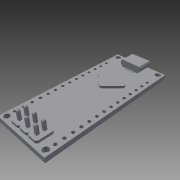
# Autodesk Inventor part: Arduino Nano
Saved by Autodesk Inventor 2015 (Build 190159000, 159)
## iProperties
Created: 2018-12-22
Part Number: Arduino Nano
Material: Типовые
Document SubType Name: Modeling
Designer: kostya
Density: 1 g/cm^3
Appearance: По умолчанию
Author: kostya
Autodesk Inventor part; units mm, degrees
ref_plane "YZ Plane" through (0, 0, 0) normal (1, 0, 0) x (0, 1, 0)
ref_plane "XZ Plane" through (0, 0, 0) normal (0, 1, 0) x (-1, 0, 0)
ref_plane "XY Plane" through (0, 0, 0) normal (0, 0, 1) x (1, 0, 0)
sketch "Эскиз1" plane through (0, 0, 0) normal (0, 0, 1) x (1, 0, 0)
  line L0 (8.9, 21.6) -> (-8.9, 21.6)
  line L1 (-8.9, 21.6) -> (-8.9, -21.6)
  line L2 (-8.9, -21.6) -> (8.9, -21.6)
  line L3 (8.9, -21.6) -> (8.9, 21.6)
  line L4 (8.9, 21.6) -> (-8.9, -21.6) construction
  line L5 (-8.9, 21.6) -> (8.9, -21.6) construction
  line L6 (8.9, 21.6) -> (7.4, 21.6) construction
  line L7 (8.9, 21.6) -> (8.9, 20.1) construction
  line L8 (7.4, 21.6) -> (8.9, 21.6) construction
  line L9 (8.9, 21.6) -> (8.9, 20.1) construction
  line L10 (8.9, 20.1) -> (7.4, 20.1) construction
  line L11 (7.4, 20.1) -> (7.4, 21.6) construction
  circle A0 centre (7.4, 20.1) radius 0.9
  line L12 (-8.9, 0) -> (8.9, 0) construction
  line L13 (0, 21.6) -> (0, -21.6) construction
  line L14 (-8.9, 20.1) -> (-7.4, 20.1) construction
  line L15 (-7.4, 20.1) -> (-7.4, 21.6) construction
  circle A1 centre (-7.4, 20.1) radius 0.9
  line L16 (8.9, -20.1) -> (7.4, -20.1) construction
  line L17 (7.4, -20.1) -> (7.4, -21.6) construction
  circle A2 centre (7.4, -20.1) radius 0.9
  circle A3 centre (-7.4, -20.1) radius 0.9
  line L18 (-8.9, -20.1) -> (-7.4, -20.1) construction
  line L19 (-7.6, 21.6) -> (7.6, 21.6) construction
  line L20 (7.6, 21.6) -> (7.6, -21.6) construction
  line L21 (7.6, -21.6) -> (-7.6, -21.6) construction
  line L22 (-7.6, -21.6) -> (-7.6, 21.6) construction
  line L23 (-7.6, 21.6) -> (7.6, -21.6) construction
  line L24 (7.6, 21.6) -> (-7.6, -21.6) construction
  line L25 (-7.6, -21.6) -> (-7.6, -17.8) construction
  circle A4 centre (-7.6, -17.8) radius 0.5
  circle A5 centre (-7.6, -15.3) radius 0.5
  circle A6 centre (-7.6, -12.8) radius 0.5
  circle A7 centre (-7.6, -10.3) radius 0.5
  circle A8 centre (-7.6, -7.8) radius 0.5
  circle A9 centre (-7.6, -5.3) radius 0.5
  circle A10 centre (-7.6, -2.8) radius 0.5
  circle A11 centre (-7.6, -0.3) radius 0.5
  circle A12 centre (-7.6, 2.2) radius 0.5
  circle A13 centre (-7.6, 4.7) radius 0.5
  circle A14 centre (-7.6, 7.2) radius 0.5
  circle A15 centre (-7.6, 9.7) radius 0.5
  circle A16 centre (-7.6, 12.2) radius 0.5
  circle A17 centre (-7.6, 14.7) radius 0.5
  line L26 (8.9, 0) -> (-8.9, 0) construction
  line L27 (7.6, -21.6) -> (7.6, 21.6) construction
  circle A18 centre (7.6, -17.8) radius 0.5
  circle A19 centre (7.6, -15.3) radius 0.5
  circle A20 centre (7.6, -12.8) radius 0.5
  circle A21 centre (7.6, -10.3) radius 0.5
  circle A22 centre (7.6, -7.8) radius 0.5
  circle A23 centre (7.6, -5.3) radius 0.5
  circle A24 centre (7.6, -2.8) radius 0.5
  circle A25 centre (7.6, -0.3) radius 0.5
  circle A26 centre (7.6, 2.2) radius 0.5
  circle A27 centre (7.6, 4.7) radius 0.5
  circle A28 centre (7.6, 7.2) radius 0.5
  circle A29 centre (7.6, 9.7) radius 0.5
  circle A30 centre (7.6, 12.2) radius 0.5
  circle A31 centre (7.6, 14.7) radius 0.5
  point P0 (0, 0)
  dimension "d0" = 17.8
  dimension "d1" = 43.2
  dimension "d2" = 1.5
  dimension "d3" = 1.5
  dimension "d4" = 1.8
  dimension "d5" = 15.2
  dimension "d6" = 3.8
  dimension "d7" = 1
  dimension "d10" = 2.5
  constraints: 56 end point, 38 symmetric about line, 32 centre point, 29 coincident, 8 midpoint, 6 parallel, 5 point on line, 3 horizontal, 3 perpendicular, 1 vertical, 56 other
  measures "d0" distance of L2.end L1.end
  measures "d1" distance of L1.end L0.end
  measures "d2" distance of L0.start L6.end
  measures "d3" distance of L0.start L7.end
  measures "d4" diameter of A0
  measures "d5" distance of L20.end L21.end
  measures "d6" distance of L21.end L25.end
  measures "d7" diameter of A4
  measures "d10" distance of A4.centre A5.centre
extrude "Выдавливание1" add sketch "Эскиз1" along normal blind 1.6
sketch "Эскиз3" plane through (0, 0, 1.6) normal (0, 0, 1) x (1, 0, 0)
  line L0 (8.9, 21.6) -> (-8.9, 21.6) construction
  line L1 (0, 21.6) -> (0, 19.5679) construction
  line L2 (0, 21.6) -> (-3.95, 21.6) construction
  line L3 (-3.95, 21.6) -> (-3.95, 16.6)
  line L4 (-3.95, 16.6) -> (0, 16.6)
  line L5 (3.95, 21.6) -> (3.95, 16.6)
  line L6 (3.95, 16.6) -> (0, 16.6)
  line L7 (-3.95, 21.6) -> (3.95, 21.6)
  point P0 (0, 0)
  dimension "d17" = 3.95
  dimension "d19" = 5
  constraints: 14 end point, 2 perpendicular, 2 symmetric about line, 2 vertical, 1 midpoint, 1 point on line
  measures "d17" distance of L1.start L2.end
  measures "d19" distance of L2.end L3.end
extrude "Выдавливание2" add sketch "Эскиз3" along normal blind 2.35
sketch "Эскиз4" plane through (-8.9, 21.6, 0) normal (0, 1, 0) x (1, 0, 0)
  line L0 (0, 0) -> (17.8, 0) projected
  line L1 (4.95, -3.95) -> (12.85, -3.95) projected
  line L2 (12.85, -1.6) -> (12.85, -3.95) projected
  line L3 (17.8, 0) -> (0, 0) projected
  line L4 (0, 0) -> (0, -1.6) projected
  line L5 (4.95, -1.6) -> (0, -1.6) projected
  line L6 (4.95, -1.6) -> (4.95, -3.95) projected
  line L7 (12.85, -3.95) -> (4.95, -3.95) projected
  line L8 (12.85, -1.6) -> (12.85, -3.95) projected
  line L9 (17.8, -1.6) -> (12.85, -1.6) projected
  line L10 (17.8, 0) -> (17.8, -1.6) projected
  line L11 (11.6, -1.6) -> (4.95, -1.6)
  line L12 (12.85, -3.95) -> (4.95, -3.95) construction
  line L13 (8.9, -1.6) -> (11.6, -1.6)
  line L14 (0, -1.6) -> (17.8, -1.6) projected
  line L15 (8.9, -3.95) -> (12, -3.95)
  line L16 (11.6, -1.6) -> (11.6, -2.35) construction
  line L17 (11.6, -1.6) -> (12.35, -2.35)
  line L18 (11.6, -1.6) -> (12.6607, -1.6) construction
  line L19 (12.35, -2.35) -> (12.35, -3.45)
  line L20 (12.35, -3.45) -> (12, -3.95)
  line L21 (8.9, -1.6) -> (6.2, -1.6)
  line L22 (8.9, -3.95) -> (5.8, -3.95)
  line L23 (6.2, -1.6) -> (5.45, -2.35)
  line L24 (5.45, -2.35) -> (5.45, -3.45)
  line L25 (5.45, -3.45) -> (5.8, -3.95)
  line L26 (11.6, -1.6) -> (12.85, -1.6) construction
  line L27 (12.85, -3.95) -> (12, -3.95) construction
  line L28 (12.85, -3.95) -> (12.85, -1.6) construction
  line L29 (4.95, -1.6) -> (4.95, -3.95) construction
  line L30 (4.95, -3.95) -> (5.8, -3.95) construction
  line L31 (12.15, -3.387) -> (12.15, -2.4328)
  line L32 (12.15, -2.4328) -> (11.5172, -1.8)
  line L33 (11.5172, -1.8) -> (8.9, -1.8)
  line L34 (8.9, -1.8) -> (6.2828, -1.8)
  line L35 (6.2828, -1.8) -> (5.65, -2.4328)
  line L36 (5.65, -2.4328) -> (5.65, -3.387)
  line L37 (5.65, -3.387) -> (5.9041, -3.75)
  line L38 (5.9041, -3.75) -> (8.9, -3.75)
  line L39 (8.9, -3.75) -> (11.8959, -3.75)
  line L40 (11.8959, -3.75) -> (12.15, -3.387)
  line L41 (8.9, -1.6) -> (8.9, -3.12) construction
  line L42 (8.9, -3.12) -> (8.9, -2.82) construction
  line L43 (7.6, -3.12) -> (10.2, -3.12)
  line L44 (10.2, -3.12) -> (10.2, -2.82)
  line L45 (7.6, -2.82) -> (7.6, -3.12)
  line L46 (7.6, -3.12) -> (10.2, -2.82) construction
  line L47 (10.2, -3.12) -> (7.6, -2.82) construction
  line L48 (10.2, -2.97) -> (7.6, -2.97) construction
  line L49 (10.2, -2.82) -> (10.1, -2.82) construction
  line L50 (10.1, -2.82) -> (9.9, -2.82) construction
  line L51 (9.9, -2.82) -> (9.9, -2.87) construction
  line L52 (9.9, -2.87) -> (10.1, -2.87) construction
  line L53 (10.1, -2.87) -> (10.1, -2.82) construction
  line L54 (10.1, -2.87) -> (9.9, -2.87)
  line L55 (9.9, -2.87) -> (9.9, -2.82)
  line L56 (9.9, -2.82) -> (10.1, -2.82)
  line L57 (10.1, -2.82) -> (10.1, -2.87)
  line L58 (10.2, -2.82) -> (10.1, -2.82)
  line L59 (9.9, -2.82) -> (7.6, -2.82)
  line L60 (9.35, -2.87) -> (9.55, -2.87) construction
  line L61 (9.55, -2.87) -> (9.55, -2.82) construction
  line L62 (9.55, -2.87) -> (9.35, -2.87)
  line L63 (9.35, -2.87) -> (9.35, -2.82)
  line L64 (9.55, -2.82) -> (9.55, -2.87)
  line L65 (8.8, -2.87) -> (9, -2.87) construction
  line L66 (9, -2.87) -> (9, -2.82) construction
  line L67 (9, -2.87) -> (8.8, -2.87)
  line L68 (8.8, -2.87) -> (8.8, -2.82)
  line L69 (9, -2.82) -> (9, -2.87)
  line L70 (8.25, -2.87) -> (8.45, -2.87) construction
  line L71 (8.45, -2.87) -> (8.45, -2.82) construction
  line L72 (8.45, -2.87) -> (8.25, -2.87)
  line L73 (8.25, -2.87) -> (8.25, -2.82)
  line L74 (8.45, -2.82) -> (8.45, -2.87)
  line L75 (7.7, -2.87) -> (7.9, -2.87) construction
  line L76 (7.9, -2.87) -> (7.9, -2.82) construction
  line L77 (7.9, -2.87) -> (7.7, -2.87)
  line L78 (7.7, -2.87) -> (7.7, -2.82)
  line L79 (7.9, -2.82) -> (7.9, -2.87)
  line L80 (9.55, -2.82) -> (9.35, -2.82)
  line L81 (9, -2.82) -> (8.8, -2.82)
  line L82 (8.45, -2.82) -> (8.25, -2.82)
  line L83 (7.9, -2.82) -> (7.7, -2.82)
  point P0 (8.9, 0)
  point P1 (8.9, -2.97)
  dimension "d22" = 2.7
  dimension "d23" = 3.1
  dimension "d24" = 0.75
  dimension "d25" = 45
  dimension "d26" = 1.1
  dimension "d28" = 0.2
  dimension "d31" = 1.52
  dimension "d32" = 0.3
  dimension "d33" = 2.6
  dimension "d38" = 0.1
  dimension "d39" = 0.2
  dimension "d40" = 0.05
  dimension "d43" = 0.55
  constraints: 142 end point, 6 horizontal, 6 midpoint, 6 parallel, 5 collinear, 5 perpendicular, 5 vertical, 4 point on line, 1 equal length, 49 other
  measures "d22" distance of L11.start L13.start
  measures "d23" distance of L15.start L15.end
  measures "d24" distance of L11.start L16.end
  measures "d25" angle of L17 L18
  measures "d26" distance of L17.end L19.end
  measures "d28" distance between parallel lines of L19 L31
  measures "d31" distance of L13.start L41.end
  measures "d32" distance of L41.end L42.end
  measures "d33" distance of L45.start L44.end
  measures "d38" distance of L49.end L44.end
  measures "d39" distance of L49.end L50.end
  measures "d40" distance of L50.end L51.end
  measures "d43" distance of L51.end L60.start
extrude "Выдавливание3" cut sketch "Эскиз4" against normal up to surface (5 mm away) contours L11 L23 L24 L25 L1 L6 | L2 L1 L20 L19 L17 L14
extrude "Выдавливание4" cut sketch "Эскиз4" against normal blind 4 contours L40 L39 L38 L37 L36 L35 L34 L33 L32 L31 | L57 L54 L55 L56
extrude "Выдавливание5" cut sketch "Эскиз4" against normal up to surface (4 mm away) contours L59 L79 L77 L78 | L59 L74 L72 L73 | L64 L62 L63 L59 | L59 L69 L67 L68
sketch "Эскиз5" plane through (0, 0, 1.6) normal (0, 0, 1) x (1, 0, 0)
  line L0 (-1.1, 16.6) -> (-1.3, 16.6)
  line L1 (-1.1, 16.6) -> (-1.1, 15.9)
  line L2 (-1.1, 15.9) -> (-1.5, 15.9)
  line L3 (-1.5, 15.9) -> (-1.5, 16.6)
  line L4 (-1.3, 16.6) -> (-1.1, 15.9) construction
  line L5 (-1.3, 16.6) -> (-1.5, 15.9) construction
  line L6 (-1.5, 16.6) -> (-1.3, 16.6)
  line L7 (-1.3, 16.6) -> (-1.1, 16.6)
  line L8 (-3.45, 16.6) -> (-2.7, 16.6) projected
  line L9 (2.7, 16.6) -> (-2.7, 16.6) projected
  line L10 (2.7, 16.6) -> (3.45, 16.6) projected
  line L11 (3.45, 16.6) -> (3.1, 16.6) projected
  line L12 (-3.1, 16.6) -> (3.1, 16.6) projected
  line L13 (-3.1, 16.6) -> (-3.45, 16.6) projected
  line L14 (-1.3, 16.6) -> (1.3, 16.6)
  line L15 (-0.45, 16.6) -> (-0.45, 15.9)
  line L16 (-0.45, 15.9) -> (-0.85, 15.9)
  line L17 (-0.85, 15.9) -> (-0.85, 16.6)
  line L18 (-0.65, 16.6) -> (-0.45, 15.9) construction
  line L19 (-0.65, 16.6) -> (-0.85, 15.9) construction
  line L20 (0.2, 16.6) -> (0.2, 15.9)
  line L21 (0.2, 15.9) -> (-0.2, 15.9)
  line L22 (-0.2, 15.9) -> (-0.2, 16.6)
  line L23 (0, 16.6) -> (0.2, 15.9) construction
  line L24 (0, 16.6) -> (-0.2, 15.9) construction
  line L25 (0.85, 16.6) -> (0.85, 15.9)
  line L26 (0.85, 15.9) -> (0.45, 15.9)
  line L27 (0.45, 15.9) -> (0.45, 16.6)
  line L28 (0.65, 16.6) -> (0.85, 15.9) construction
  line L29 (0.65, 16.6) -> (0.45, 15.9) construction
  line L30 (1.5, 16.6) -> (1.5, 15.9)
  line L31 (1.5, 15.9) -> (1.1, 15.9)
  line L32 (1.1, 15.9) -> (1.1, 16.6)
  line L33 (1.3, 16.6) -> (1.5, 15.9) construction
  line L34 (1.3, 16.6) -> (1.1, 15.9) construction
  line L35 (-1.5, 16.6) -> (1.5, 16.6)
  line L36 (-1.5, 16.6) -> (-1.1, 16.6)
  line L37 (2.7, 16.6) -> (-2.7, 16.6) projected
  line L38 (-0.85, 16.6) -> (-0.45, 16.6)
  line L39 (-0.2, 16.6) -> (0.2, 16.6)
  line L40 (0.45, 16.6) -> (0.85, 16.6)
  line L41 (1.1, 16.6) -> (1.5, 16.6)
  point P0 (0, 0)
  dimension "d52" = 0.4
  dimension "d54" = 2.6
  dimension "d57" = 0.65
  constraints: 80 end point, 6 collinear, 2 horizontal, 1 parallel, 1 point on line, 40 other
  measures "d52" distance of L1.end L2.end
  measures "d54" distance of L0.end L14.end
  measures "d57" distance of L2.end L17.start
extrude "Выдавливание6" add sketch "Эскиз5" along normal blind 0.1
sketch "Эскиз6" plane through (0, 0, 1.6) normal (0, 0, 1) x (1, 0, 0)
  circle A0 centre (7.4, -20.1) radius 0.9 projected
  circle A1 centre (-7.4, -20.1) radius 0.9 projected
  circle A2 centre (-7.4, 20.1) radius 0.9 projected
  circle A3 centre (7.4, 20.1) radius 0.9 projected
  circle A4 centre (7.6, 12.2) radius 0.5 projected
  circle A5 centre (7.6, 14.7) radius 0.5 projected
  circle A6 centre (7.6, 9.7) radius 0.5 projected
  circle A7 centre (7.6, 7.2) radius 0.5 projected
  circle A8 centre (7.6, 4.7) radius 0.5 projected
  circle A9 centre (7.6, 2.2) radius 0.5 projected
  circle A10 centre (7.6, -0.3) radius 0.5 projected
  circle A11 centre (7.6, -2.8) radius 0.5 projected
  circle A12 centre (7.6, -5.3) radius 0.5 projected
  circle A13 centre (7.6, -7.8) radius 0.5 projected
  circle A14 centre (7.6, -12.8) radius 0.5 projected
  circle A15 centre (7.6, -10.3) radius 0.5 projected
  circle A16 centre (7.6, -15.3) radius 0.5 projected
  circle A17 centre (7.6, -17.8) radius 0.5 projected
  circle A18 centre (-7.6, 14.7) radius 0.5 projected
  circle A19 centre (-7.6, 12.2) radius 0.5 projected
  circle A20 centre (-7.6, 9.7) radius 0.5 projected
  circle A21 centre (-7.6, 7.2) radius 0.5 projected
  circle A22 centre (-7.6, 4.7) radius 0.5 projected
  circle A23 centre (-7.6, 2.2) radius 0.5 projected
  circle A24 centre (-7.6, -0.3) radius 0.5 projected
  circle A25 centre (-7.6, -2.8) radius 0.5 projected
  circle A26 centre (-7.6, -5.3) radius 0.5 projected
  circle A27 centre (-7.6, -7.8) radius 0.5 projected
  circle A28 centre (-7.6, -10.3) radius 0.5 projected
  circle A29 centre (-7.6, -12.8) radius 0.5 projected
  circle A30 centre (-7.6, -15.3) radius 0.5 projected
  circle A31 centre (-7.6, -17.8) radius 0.5 projected
  line L0 (0.85, 16.6) -> (0.85, 15.9) projected
  line L1 (0.85, 15.9) -> (0.45, 15.9) projected
  line L2 (0.45, 15.9) -> (0.45, 16.6) projected
  line L3 (0.45, 16.6) -> (0.2, 16.6) projected
  line L4 (0.2, 16.6) -> (0.2, 15.9) projected
  line L5 (0.2, 15.9) -> (-0.2, 15.9) projected
  line L6 (-0.2, 15.9) -> (-0.2, 16.6) projected
  line L7 (-0.2, 16.6) -> (-0.45, 16.6) projected
  line L8 (-0.45, 16.6) -> (-0.45, 15.9) projected
  line L9 (-0.45, 15.9) -> (-0.85, 15.9) projected
  line L10 (-0.85, 15.9) -> (-0.85, 16.6) projected
  line L11 (-0.85, 16.6) -> (-1.1, 16.6) projected
  line L12 (-1.1, 16.6) -> (-1.1, 15.9) projected
  line L13 (-1.1, 15.9) -> (-1.5, 15.9) projected
  line L14 (-1.5, 15.9) -> (-1.5, 16.6) projected
  line L15 (-1.5, 16.6) -> (-2.7, 16.6) projected
  line L16 (-2.7, 21.6) -> (-2.7, 16.6) projected
  line L17 (-2.7, 21.6) -> (-8.9, 21.6) projected
  line L18 (-8.9, 21.6) -> (-8.9, -21.6) projected
  line L19 (-8.9, -21.6) -> (8.9, -21.6) projected
  line L20 (8.9, -21.6) -> (8.9, 21.6) projected
  line L21 (8.9, 21.6) -> (2.7, 21.6) projected
  line L22 (2.7, 16.6) -> (2.7, 21.6) projected
  line L23 (2.7, 16.6) -> (1.5, 16.6) projected
  line L24 (1.5, 16.6) -> (1.5, 15.9) projected
  line L25 (1.5, 15.9) -> (1.1, 15.9) projected
  line L26 (1.1, 15.9) -> (1.1, 16.6) projected
  line L27 (1.1, 16.6) -> (0.85, 16.6) projected
  line L28 (-8.9, -21.6) -> (8.9, -21.6) construction
  line L29 (0, -21.6) -> (0, 8.4) construction
  line L30 (0, 8.4) -> (0, 3.4) construction
  line L31 (0, 8.4) -> (0, 13.4) construction
  line L32 (0.3536, 13.0464) -> (4.6464, 8.7536)
  line L33 (4.6464, 8.0464) -> (0.3536, 3.7536)
  line L34 (-0.3536, 3.7536) -> (-4.6464, 8.0464)
  line L35 (-4.6464, 8.7536) -> (-0.3536, 13.0464)
  line L36 (-0.3536, 3.7536) -> (0.3536, 3.7536)
  line L37 (-0.3536, 13.0464) -> (0.3536, 13.0464)
  line L38 (-4.6464, 8.7536) -> (-4.6464, 8.0464)
  line L39 (4.6464, 8.7536) -> (4.6464, 8.0464)
  point P0 (0, 0)
  dimension "d64" = 30
  dimension "d65" = 5
  dimension "d66" = 5
  constraints: 22 end point, 3 vertical, 2 horizontal, 1 coincident, 1 midpoint, 1 parallel, 1 point on line, 5 other
  measures "d64" distance of L29.start L29.end
  measures "d65" distance of L29.end L30.end
  measures "d66" distance of L29.end L31.end
extrude "Выдавливание7" add sketch "Эскиз6" along normal blind 0.7 contours L32 L39 L33 L36 L34 L38 L35 L37
sketch "Эскиз7" plane through (0, 0, 1.6) normal (0, 0, 1) x (1, 0, 0)
  line L0 (4.6464, 8.7536) -> (4.6464, 8.0464) projected
  line L1 (4.6464, 8.0464) -> (0.3536, 3.7536) projected
  line L2 (0.3536, 3.7536) -> (-0.3536, 3.7536) projected
  line L3 (-0.3536, 3.7536) -> (-4.6464, 8.0464) projected
  line L4 (-4.6464, 8.0464) -> (-4.6464, 8.7536) projected
  line L5 (-4.6464, 8.7536) -> (-0.3536, 13.0464) projected
  line L6 (-0.3536, 13.0464) -> (0.3536, 13.0464) projected
  line L7 (0.3536, 13.0464) -> (4.6464, 8.7536) projected
  circle A0 centre (7.4, -20.1) radius 0.9 projected
  circle A1 centre (-7.4, -20.1) radius 0.9 projected
  circle A2 centre (-7.4, 20.1) radius 0.9 projected
  circle A3 centre (7.4, 20.1) radius 0.9 projected
  circle A4 centre (7.6, 12.2) radius 0.5 projected
  circle A5 centre (7.6, 14.7) radius 0.5 projected
  circle A6 centre (7.6, 9.7) radius 0.5 projected
  circle A7 centre (7.6, 7.2) radius 0.5 projected
  circle A8 centre (7.6, 4.7) radius 0.5 projected
  circle A9 centre (7.6, 2.2) radius 0.5 projected
  circle A10 centre (7.6, -0.3) radius 0.5 projected
  circle A11 centre (7.6, -2.8) radius 0.5 projected
  circle A12 centre (7.6, -5.3) radius 0.5 projected
  circle A13 centre (7.6, -7.8) radius 0.5 projected
  circle A14 centre (7.6, -12.8) radius 0.5 projected
  circle A15 centre (7.6, -10.3) radius 0.5 projected
  circle A16 centre (7.6, -15.3) radius 0.5 projected
  circle A17 centre (7.6, -17.8) radius 0.5 projected
  circle A18 centre (-7.6, 14.7) radius 0.5 projected
  circle A19 centre (-7.6, 12.2) radius 0.5 projected
  circle A20 centre (-7.6, 9.7) radius 0.5 projected
  circle A21 centre (-7.6, 7.2) radius 0.5 projected
  circle A22 centre (-7.6, 4.7) radius 0.5 projected
  circle A23 centre (-7.6, 2.2) radius 0.5 projected
  circle A24 centre (-7.6, -0.3) radius 0.5 projected
  circle A25 centre (-7.6, -2.8) radius 0.5 projected
  circle A26 centre (-7.6, -5.3) radius 0.5 projected
  circle A27 centre (-7.6, -7.8) radius 0.5 projected
  circle A28 centre (-7.6, -10.3) radius 0.5 projected
  circle A29 centre (-7.6, -12.8) radius 0.5 projected
  circle A30 centre (-7.6, -15.3) radius 0.5 projected
  circle A31 centre (-7.6, -17.8) radius 0.5 projected
  line L8 (0.85, 16.6) -> (0.85, 15.9) projected
  line L9 (0.85, 15.9) -> (0.45, 15.9) projected
  line L10 (0.45, 15.9) -> (0.45, 16.6) projected
  line L11 (0.45, 16.6) -> (0.2, 16.6) projected
  line L12 (0.2, 16.6) -> (0.2, 15.9) projected
  line L13 (0.2, 15.9) -> (-0.2, 15.9) projected
  line L14 (-0.2, 15.9) -> (-0.2, 16.6) projected
  line L15 (-0.2, 16.6) -> (-0.45, 16.6) projected
  line L16 (-0.45, 16.6) -> (-0.45, 15.9) projected
  line L17 (-0.45, 15.9) -> (-0.85, 15.9) projected
  line L18 (-0.85, 15.9) -> (-0.85, 16.6) projected
  line L19 (-0.85, 16.6) -> (-1.1, 16.6) projected
  line L20 (-1.1, 16.6) -> (-1.1, 15.9) projected
  line L21 (-1.1, 15.9) -> (-1.5, 15.9) projected
  line L22 (-1.5, 15.9) -> (-1.5, 16.6) projected
  line L23 (-1.5, 16.6) -> (-2.7, 16.6) projected
  line L24 (-2.7, 21.6) -> (-2.7, 16.6) projected
  line L25 (-2.7, 21.6) -> (-8.9, 21.6) projected
  line L26 (-8.9, 21.6) -> (-8.9, -21.6) projected
  line L27 (-8.9, -21.6) -> (8.9, -21.6) projected
  line L28 (8.9, -21.6) -> (8.9, 21.6) projected
  line L29 (8.9, 21.6) -> (2.7, 21.6) projected
  line L30 (2.7, 16.6) -> (2.7, 21.6) projected
  line L31 (2.7, 16.6) -> (1.5, 16.6) projected
  line L32 (1.5, 16.6) -> (1.5, 15.9) projected
  line L33 (1.5, 15.9) -> (1.1, 15.9) projected
  line L34 (1.1, 15.9) -> (1.1, 16.6) projected
  line L35 (1.1, 16.6) -> (0.85, 16.6) projected
  line L36 (-8.9, -21.6) -> (8.9, -21.6) construction
  line L37 (-5, -16.1) -> (-5, -20.1)
  line L38 (-4.5, -15.6) -> (-2.2, -15.6)
  line L39 (-8.9, -21.6) -> (8.9, -21.6) projected
  line L40 (-4.5, -15.6) -> (-2.2, -15.6)
  line L41 (-1.7, -16.1) -> (-1.7, -20.1)
  line L42 (-2.2, -20.6) -> (-4.5, -20.6)
  line L43 (-5, -20.1) -> (-5, -16.1)
  line L44 (-4.5, -20.6) -> (-2.2, -20.6)
  line L45 (-2.2, -15.6) -> (-4.5, -15.6)
  line L46 (-5, -20.1) -> (-4.5, -20.6)
  line L47 (-2.2, -20.6) -> (-1.7, -20.1)
  line L48 (-2.2, -15.6) -> (-1.7, -16.1)
  line L49 (-4.5, -15.6) -> (-5, -16.1)
  line L50 (-3.35, -18.1) -> (-3.35, -20.6) construction
  line L51 (-1.7, -18.1) -> (-5, -18.1) construction
  line L52 (-3.35, -21.6) -> (-3.35, -20.6) construction
  point P0 (0, 0)
  dimension "d91" = 1
  constraints: 30 end point, 4 midpoint, 4 perpendicular, 3 parallel, 2 horizontal, 1 point on line
  measures "d91" distance of L52.start L50.end
extrude "Выдавливание8" add sketch "Эскиз7" along normal blind 0.8 contours L49 L38 L48 L41 L47 L42 L46 L37
sketch "Эскиз8" plane through (0, 0, 2.4) normal (0, 0, 1) x (1, 0, 0)
  line L0 (-4.5, -20.6) -> (-2.2, -20.6) projected
  line L1 (-2.2, -20.6) -> (-1.7, -20.1) projected
  line L2 (-1.7, -20.1) -> (-1.7, -16.1) projected
  line L3 (-1.7, -16.1) -> (-2.2, -15.6) projected
  line L4 (-2.2, -15.6) -> (-4.5, -15.6) projected
  line L5 (-4.5, -15.6) -> (-5, -16.1) projected
  line L6 (-5, -16.1) -> (-5, -20.1) projected
  line L7 (-5, -20.1) -> (-4.5, -20.6) projected
  line L8 (-5, -18.1) -> (-1.7, -18.1) construction
  line L9 (-5, -16.1) -> (-1.7, -16.1) construction
  line L10 (-1.7, -20.1) -> (-5, -20.1) construction
  line L11 (-3.35, -15.6) -> (-3.35, -16.1) construction
  line L12 (-3.35, -16.1) -> (-3.35, -18.1) construction
  line L13 (-3.35, -20.1) -> (-3.35, -20.6) construction
  line L14 (-4.5, -20.6) -> (-2.2, -20.6) construction
  line L15 (-3.75, -16.7) -> (-2.95, -16.7)
  line L16 (-2.95, -16.7) -> (-2.95, -17.5)
  line L17 (-2.95, -17.5) -> (-3.75, -17.5)
  line L18 (-3.75, -17.5) -> (-3.75, -16.7)
  line L19 (-3.75, -16.7) -> (-2.95, -17.5) construction
  line L20 (-2.95, -16.7) -> (-3.75, -17.5) construction
  line L21 (-3.35, -20.1) -> (-3.35, -18.1) construction
  line L22 (-3.75, -19.5) -> (-2.95, -19.5)
  line L23 (-2.95, -19.5) -> (-2.95, -18.7)
  line L24 (-2.95, -18.7) -> (-3.75, -18.7)
  line L25 (-3.75, -18.7) -> (-3.75, -19.5)
  line L26 (-3.75, -19.5) -> (-2.95, -18.7) construction
  line L27 (-2.95, -19.5) -> (-3.75, -18.7) construction
  point P0 (0, 0)
  point P1 (-3.35, -17.1)
  point P2 (-3.35, -19.1)
  dimension "d98" = 0.8
  dimension "d99" = 0.8
  constraints: 38 end point, 12 midpoint, 5 symmetric about line, 3 parallel, 2 horizontal, 1 perpendicular
  measures "d98" distance of L16.end L17.end
  measures "d99" distance of L15.end L16.end
extrude "Выдавливание9" add sketch "Эскиз8" along normal blind 3 contours L15 L16 L17 L18 | L25 L24 L23 L22
pattern_linear "Прямоуг.массив1" count 3 spacing 3.3 along (1, 0, 0) of "Выдавливание8", "Выдавливание9"
chamfer "Фаска1" distance 0.25 angle 45 24 edges at (-3.35, -19.5, 5.4) (-2.95, -19.1, 5.4) (-3.35, -18.7, 5.4) (-3.75, -19.1, 5.4) (-2.95, -17.1, 5.4) (-3.35, -17.5, 5.4) (-3.75, -17.1, 5.4) (-3.35, -16.7, 5.4) (0.35, -17.1, 5.4) (-0.05, -17.5, 5.4) (-0.45, -17.1, 5.4) (-0.05, -16.7, 5.4) (0.35, -19.1, 5.4) (-0.05, -19.5, 5.4) (-0.45, -19.1, 5.4) (-0.05, -18.7, 5.4) (2.85, -19.1, 5.4) (3.25, -19.5, 5.4) (3.65, -19.1, 5.4) (3.25, -18.7, 5.4) (3.65, -17.1, 5.4) (3.25, -17.5, 5.4) (2.85, -17.1, 5.4) (3.25, -16.7, 5.4)
